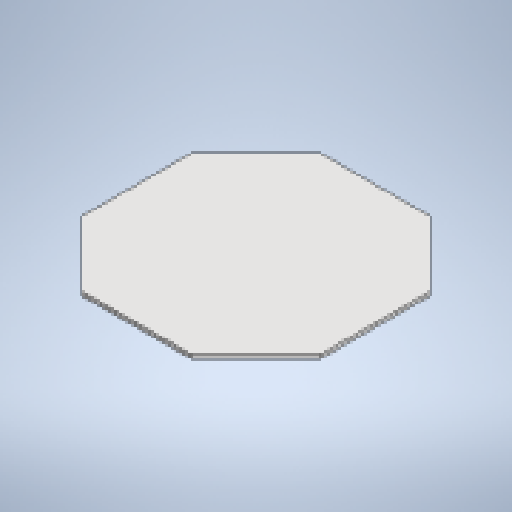
# Autodesk Inventor part: DSB 210 Axis cap
Saved by Autodesk Inventor 2025.1 (Build 291241020, 241B)
## iProperties
Created: 2024-12-09
Part Number: DSB 210 Axis cap
Material: Stainless Steel
Document SubType Name: Sheet Metal
Designer: admin
Mass: 344.52 g
Surface Area: 230.435 cm^2
Volume: 43.065 cm^3
Density: 8 g/cm^3
Flat Pattern Width: 19.7 cm
Flat Pattern Length: 19.7 cm
Flat Pattern Area: 388.09 cm^2
Sheet Metal Rule: AISI304 3mm Die 32
Sheet Metal Width: 197.000 mm
Sheet Metal Length: 197.000 mm
Sheet Metal Area: 38809.000 mm^2
Appearance: Default
Author: user
Autodesk Inventor part; units mm, degrees
ref_plane "YZ Plane" through (0, 0, 0) normal (1, 0, 0) x (0, 1, 0)
ref_plane "XZ Plane" through (0, 0, 0) normal (0, 1, 0) x (-1, 0, 0)
ref_plane "XY Plane" through (0, 0, 0) normal (0, 0, 1) x (1, 0, 0)
sketch "Sketch8" plane through (0, 0, 0) normal (0, 0, 1) x (1, 0, 0)
  line L0 (98.5, -98.5) -> (-98.5, -98.5)
  line L1 (-98.5, -98.5) -> (-98.5, 98.5)
  line L2 (-98.5, 98.5) -> (98.5, 98.5)
  line L3 (98.5, 98.5) -> (98.5, -98.5)
  line L4 (98.5, -98.5) -> (-98.5, 98.5) construction
  line L5 (-98.5, -98.5) -> (98.5, 98.5) construction
  line L6 (45, -98.5) -> (98.5, -45)
  line L7 (-45, -98.5) -> (-98.5, -45)
  line L8 (98.5, 45) -> (45, 98.5)
  line L9 (-45, 98.5) -> (-98.5, 45)
  line L10 (0, -98.5) -> (0, 98.5) construction
  point P0 (0, 0)
  dimension "d42" = 197
  dimension "d43" = 197
  dimension "d44" = 90
  measures "d42" distance of L0.start L0.end
  measures "d43" distance of L0.end L1.end
  measures "d44" distance of L7.start L6.start
extrude "Plate3" add sketch "Sketch8" along normal blind 3 contours L0 L7 L1 L9 L2 L8 L3 L6
fillet "Corner Round1" radius 6 8 edges at (-45, -98.5, 1.5) (45, -98.5, 1.5) (98.5, -45, 1.5) (98.5, 45, 1.5) (45, 98.5, 1.5) (-45, 98.5, 1.5) (-98.5, 45, 1.5) (-98.5, -45, 1.5)
equation "\"d43\" = d42"
equation "\"d45\" = Thickness"
equation "\"BendReliefWidth\" = Thickness"
equation "\"BendReliefDepth\" = 0.5 * Thickness"
equation "\"CornerReliefSize\" = 4 * Thickness"
equation "\"MinimumRemnant\" = 2 * Thickness"
equation "\"TransitionRadius\" = BendRadius"
equation "\"JacobiRadiusSize\" = BendRadius"
equation "\"GapSize\" = Thickness"
equation "\"Thickness\" = 3"
equation "\"BendRadius\" = 5"
body "Solid2"
